# Autodesk Inventor part: SingleCrank
Saved by Autodesk Inventor 2011 SP2 (Build 150309200, 309)
## iProperties
Created: 2014-05-26
Part Number: SingleCrank
Document SubType Name: Modeling
Designer: Maurice Woods
Density: 1 g/cm^3
Author: Maurice Woods
Autodesk Inventor part; units mm, degrees
ref_plane "YZ Plane" through (0, 0, 0) normal (1, 0, 0) x (0, 1, 0)
ref_plane "XZ Plane" through (0, 0, 0) normal (0, 1, 0) x (-1, 0, 0)
ref_plane "XY Plane" through (0, 0, 0) normal (0, 0, 1) x (1, 0, 0)
sketch "Sketch1" plane through (0, 0, 0) normal (0, 0, 1) x (1, 0, 0)
  line L0 (1.6483, 5.0443) -> (1.6483, 5.0443)
  line L1 (5.6483, 1.0443) -> (5.6483, -8.9821)
  line L2 (1.6483, -12.9821) -> (1.6483, -12.9821)
  line L3 (-2.3517, -8.9821) -> (-2.3517, 1.0443)
  arc A0 (1.6483, -12.9821) -> (5.6483, -8.9821) centre (1.6483, -8.9821) ccw
  arc A1 (-2.3517, -8.9821) -> (1.6483, -12.9821) centre (1.6483, -8.9821) ccw
  arc A2 (1.6483, 5.0443) -> (-2.3517, 1.0443) centre (1.6483, 1.0443) ccw
  arc A3 (5.6483, 1.0443) -> (1.6483, 5.0443) centre (1.6483, 1.0443) ccw
  point P0 (0, 0)
  point P1 (5.6483, -12.9821)
  point P2 (-2.3517, -12.9821)
  dimension "d0" = 8
  dimension "d1" = 4
  dimension "d2" = 10.0263
  constraints: 8 end point, 8 point on circle, 8 tangent, 4 centre point, 4 point on line, 3 equal radius, 2 parallel, 1 horizontal, 1 perpendicular
  measures "d0" distance of point (5.648, -12.982) point (-2.352, -12.982)
  measures "d1" radius of A0
  measures "d2" distance of A0.centre A2.centre
extrude "Extrusion1" add sketch "Sketch1" along normal blind 5
equation "\"d2\" = LengthM"
equation "\"LengthM\" = 10.02632"
body "Solid1"
